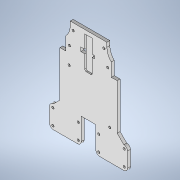
# Autodesk Inventor part: Основа робота
Saved by Autodesk Inventor 2020 (Build 240168000, 168)
## iProperties
Created: 2021-02-28
Part Number: Основа робота
Material: Типовые
Document SubType Name: Обычные детали
Designer: Антон
Density: 1 g/cm^3
Appearance: По умолчанию
Mass: 52.0111 g
Surface Area: 352.197 cm^2
Volume: 52.0111 cm^3
Sheet Metal Rule: По умолчанию
Author: Антон
Autodesk Inventor part; units mm, degrees
note: some values were not read from the file. Chosen so that the rebuilt part matches the saved one: direction of "Рельеф1".
ref_plane "YZ Plane" through (0, 0, 0) normal (1, 0, 0) x (0, 1, 0)
ref_plane "XZ Plane" through (0, 0, 0) normal (0, 1, 0) x (-1, 0, 0)
ref_plane "XY Plane" through (0, 0, 0) normal (0, 0, 1) x (1, 0, 0)
sketch "Эскиз1" plane through (0, 0, 0) normal (0, 0, 1) x (1, 0, 0)
  line L0 (0, 0) -> (39, 0)
  line L1 (39, 0) -> (39, 139.6)
  line L2 (39, 139.6) -> (0, 139.6)
  line L3 (0, 139.6) -> (0, 0)
  line L4 (0, 0) -> (-14.05, 0)
  line L5 (-14.05, 0) -> (-14.05, 30.3)
  line L6 (-14.05, 30.3) -> (0, 30.3)
  line L7 (0, 30.3) -> (0, 0)
  line L8 (-14.05, 0) -> (-9.5, 0)
  line L9 (-9.5, 0) -> (-9.5, 4.55)
  line L10 (-9.5, 4.55) -> (-9.5, 25.75)
  circle A0 centre (-9.5, 25.75) radius 1.6
  circle A1 centre (-9.5, 4.55) radius 1.6
  line L11 (39, 0) -> (29, 0)
  line L12 (29, 0) -> (29, 35)
  line L13 (29, 35) -> (39, 35)
  line L14 (39, 35) -> (39, 0)
  line L15 (29, 4.55) -> (25, 4.55)
  line L16 (29, 25.75) -> (25, 25.75)
  circle A2 centre (25, 25.75) radius 1.6
  circle A3 centre (25, 4.55) radius 1.6
  line L17 (39, 139.6) -> (39, 130.4)
  line L18 (39, 130.4) -> (18, 130.4)
  circle A4 centre (18, 130.4) radius 1.6
  line L19 (39, 139.6) -> (34, 139.6)
  line L20 (34, 139.6) -> (18, 139.6)
  line L21 (25, 25.75) -> (25, 4.55)
  circle A5 centre (12.95, 110.25) radius 1.6
  line L22 (0, 139.6) -> (14, 139.6)
  line L23 (14, 139.6) -> (14, 119.25)
  line L24 (14, 119.25) -> (0, 119.25)
  line L25 (0, 119.25) -> (0, 139.6)
  line L26 (0, 119.25) -> (8, 119.25)
  line L27 (8, 119.25) -> (8, 101.25)
  line L28 (8, 101.25) -> (0, 101.25)
  line L29 (0, 101.25) -> (0, 119.25)
  point P0 (0, 30.3)
  point P1 (29, 0)
  point P2 (39, 35)
  point P3 (0, 182.1)
  point P4 (25, 15.15)
  point P5 (-9.5, 15.15)
  point P6 (0, 119.25)
  point P7 (8, 119.25)
  point P8 (0, 101.25)
  dimension "d0" = 39
  dimension "d1" = 139.6
  dimension "d191" = 14.05
  dimension "d192" = 30.3
  dimension "d207" = 4.55
  dimension "d208" = 4.55
  dimension "d209" = 21.2
  dimension "d210" = 10
  dimension "d211" = 35
  dimension "d215" = 4
  dimension "d290" = 3.2
  dimension "d309" = 21
  dimension "d311" = 3.2
  dimension "d325" = 9.2
  dimension "d387" = 21.2
  dimension "d418" = 4.55
  dimension "d419" = 12.95
  dimension "d420" = 29.35
  dimension "d421" = 3.2
  dimension "d424" = 14
  dimension "d425" = 20.35
  dimension "d427" = 8
  dimension "d428" = 18
  constraints: 60 end point, 11 parallel, 8 perpendicular, 7 horizontal, 6 centre point, 6 point on line, 5 coincident, 3 equal radius, 2 midpoint, 1 collinear, 1 horizontal alignment, 1 vertical
  measures "d0" distance of L2.end L1.end
  measures "d1" distance of L1.end L0.end
  measures "d191" distance of L5.end L6.end
  measures "d192" distance of L4.end L5.end
  measures "d207" distance of L4.end L8.end
  measures "d208" distance of L8.end L9.end
  measures "d209" distance of L9.end L10.end
  measures "d210" distance of L12.end L13.end
  measures "d211" distance of L11.end L12.end
  measures "d215" distance of L16.start L16.end
  measures "d290" diameter of A2
  measures "d309" distance of L17.end L18.end
  measures "d311" diameter of A4
  measures "d325" distance from line of L19.end L18
  measures "d387" distance of L21.end L21.start
  measures "d418" distance from line of L0 L15.end
  measures "d419" distance from line of L3 A5.centre
  measures "d420" distance from line of L2 A5.centre
  measures "d421" diameter of A5
  measures "d424" distance of L23.end L24.end
  measures "d425" distance of L22.end L23.end
  measures "d427" distance of L27.end L28.end
  measures "d428" distance of L26.end L27.end
extrude "Выдавливание1" add sketch "Эскиз1" along normal blind 4 contours L3 L28 L27 L24 L23 L2 L1 L13 L12 L16 A2 L21 A3 L15 L0 | L4 L5 L6 L3 | L15 A3 L21 A2 L16 L12
mirror "Зеркальное отражение1" about plane through (39, 35, 0) normal (1, 0, 0) of "Выдавливание1"
sketch "Эскиз18" plane through (0, 0, 4) normal (0, 0, 1) x (1, 0, 0)
  line L0 (39, 139.6) -> (39, 86.75)
  line L1 (39, 86.75) -> (12.6, 86.75)
  line L2 (39, 86.75) -> (39, 41.05)
  line L3 (39, 41.05) -> (67.8, 41.05)
  line L4 (14, 139.6) -> (64, 139.6) projected
  point P0 (-4.55, 159.6)
  point P1 (82.55, 159.6)
  point P2 (0, 139.6)
  point P3 (78, 139.6)
  dimension "d218" = 52.85
  dimension "d220" = 26.4
  dimension "d221" = 45.7
  dimension "d222" = 28.8
  constraints: 8 end point, 2 horizontal, 2 vertical, 2 other
  measures "d218" distance of L0.start L0.end
  measures "d220" distance of L0.end L1.end
  measures "d221" distance of L0.end L2.end
  measures "d222" distance of L2.end L3.end
hole "Отверстие10" at (12.6, 86.75, 4) at (67.8, 41.05, 4) direction (0, 0, -1) diameter 3.2 end through all
fillet "Сопряжение2" radius 5.05 6 edges at (-14.05, 30.3, 2) (-14.05, 0, 2) (29, 0, 2) (49, 0, 2) (92.05, 0, 2) (92.05, 30.3, 2)
sketch "Эскиз19" plane through (0, 0, 0) normal (0, 0, -1) x (-1, 0, 0)
  line L0 (-14, 139.6) -> (-64, 139.6) projected
  circle A0 centre (-12.6, 86.75) radius 1.6 projected
  circle A1 centre (-12.6, 86.75) radius 1.6 projected
  line L1 (-15.4, 88.3666) -> (-12.6, 89.9832)
  line L2 (-12.6, 89.9832) -> (-9.8, 88.3666)
  line L3 (-9.8, 88.3666) -> (-9.8, 85.1334)
  line L4 (-9.8, 85.1334) -> (-12.6, 83.5168)
  line L5 (-12.6, 83.5168) -> (-15.4, 85.1334)
  line L6 (-15.4, 85.1334) -> (-15.4, 88.3666)
  line L7 (0, 101.25) -> (0, 30.3) projected
  point P0 (0, 139.6)
  point P1 (-78, 139.6)
  point P2 (0, 119.25)
  dimension "d423" = 5.6
  constraints: 12 end point, 1 coincident, 1 parallel, 13 other
  measures "d423" distance between parallel lines of L3 L6
extrude "Выдавливание7" cut sketch "Эскиз19" against normal blind 2.6 contours A0 | L1 L2 L3 L4 L5 L6
chamfer "Фаска1" distance 9 angle 45 2 edges at (0, 30.3, 2) (78, 30.3, 2)
sketch "Эскиз21" plane through (0, 0, 4) normal (0, 0, 1) x (1, 0, 0)
  line L0 (39, 139.6) -> (39, 134.4)
  line L1 (44.05, 134.4) -> (33.95, 134.4)
  line L2 (33.95, 134.4) -> (33.95, 90.75)
  line L3 (33.95, 90.75) -> (44.05, 90.75)
  line L4 (44.05, 90.75) -> (44.05, 134.4)
  line L5 (42, 92.8) -> (36, 92.8) construction
  line L6 (42, 90.75) -> (36, 90.75)
  line L7 (36, 94.85) -> (42, 94.85)
  arc A0 (42, 90.75) -> (42, 94.85) centre (42, 92.8) ccw
  arc A1 (36, 94.85) -> (36, 90.75) centre (36, 92.8) ccw
  line L8 (14, 139.6) -> (64, 139.6) projected
  point P0 (0, 0)
  point P1 (39, 92.8)
  point P2 (33.95, 92.8)
  point P3 (42, 90.75)
  point P4 (44.05, 92.8)
  point P5 (-4.55, 159.6)
  point P6 (82.55, 159.6)
  point P7 (0, 139.6)
  point P8 (78, 139.6)
  dimension "d297" = 10.1
  dimension "d298" = 43.65
  dimension "d299" = 5.2
  dimension "d307" = 4.1
  constraints: 18 end point, 6 tangent, 4 point on circle, 3 parallel, 2 centre point, 2 midpoint, 2 perpendicular, 1 collinear, 1 horizontal, 1 vertical, 2 other
  measures "d297" distance of L3.end L2.end
  measures "d298" distance of L2.end L1.end
  measures "d299" distance of L0.start L0.end
  measures "d307" distance between parallel lines of L3 L7
extrude "Выдавливание9" cut sketch "Эскиз21" against normal blind 2 contours L4 A0 L7 A1 L2 L1 | A0 L3 A1 L7
sketch "Эскиз25" plane through (0, 0, 0) normal (0, 0, -1) x (-1, 0, 0)
  circle A0 centre (-25, 25.75) radius 1.6 projected
  circle A1 centre (-25, 4.55) radius 1.6 projected
  circle A2 centre (9.5, 25.75) radius 1.6 projected
  circle A3 centre (9.5, 4.55) radius 1.6 projected
  circle A4 centre (-53, 25.75) radius 1.6 projected
  circle A5 centre (-53, 4.55) radius 1.6 projected
  circle A6 centre (-87.5, 4.55) radius 1.6 projected
  circle A7 centre (-87.5, 25.75) radius 1.6 projected
  circle A8 centre (-67.8, 41.05) radius 1.6 projected
  circle A9 centre (-12.6, 86.75) radius 1.6 projected
  circle A10 centre (-18, 130.4) radius 1.6 projected
  circle A11 centre (-60, 130.4) radius 1.6 projected
  circle A12 centre (-65.05, 110.25) radius 1.6 projected
  circle A13 centre (-12.95, 110.25) radius 1.6 projected
  circle A14 centre (-65.05, 110.25) radius 1.6 projected
  circle A15 centre (-12.95, 110.25) radius 1.6 projected
  point P0 (0, 0)
  constraints: 14 coincident
pattern_sketch "Массив по эскизу1" of "Выдавливание7" from (12.6, 86.75, 0) copies at (25, 25.75, 0) at (25, 4.55, 0) at (-9.5, 25.75, 0) at (-9.5, 4.55, 0) at (53, 25.75, 0) at (53, 4.55, 0) at (87.5, 4.55, 0) at (87.5, 25.75, 0) at (67.8, 41.05, 0) at (18, 130.4, 0) at (60, 130.4, 0) at (65.05, 110.25, 0) at (12.95, 110.25, 0)
sketch "Эскиз29" plane through (0, 0, 4) normal (0, 0, 1) x (1, 0, 0)
  line L0 (47.05, 111.6) -> (44.05, 111.6)
  line L1 (44.05, 111.6) -> (44.05, 115.6)
  line L2 (44.05, 115.6) -> (47.05, 115.6)
  line L3 (47.05, 115.6) -> (47.05, 111.6)
  line L4 (44.05, 134.4) -> (44.05, 92.8) projected
  line L5 (33.95, 110.85) -> (28.45, 110.85)
  line L6 (28.45, 110.85) -> (28.45, 116.35)
  line L7 (28.45, 116.35) -> (33.95, 116.35)
  line L8 (33.95, 116.35) -> (33.95, 110.85)
  line L9 (33.95, 92.8) -> (33.95, 134.4) projected
  point P0 (0, 0)
  point P1 (44.05, 113.6)
  point P2 (44.05, 136.615)
  point P3 (33.95, 113.6)
  point P4 (33.95, 136.615)
  dimension "d405" = 3
  dimension "d406" = 4
  dimension "d407" = 5.5
  dimension "d408" = 5.5
  constraints: 16 end point, 4 midpoint, 4 parallel, 2 horizontal, 2 perpendicular
  measures "d405" distance of L1.end L2.end
  measures "d406" distance of L0.end L1.end
  measures "d407" distance of L5.start L5.end
  measures "d408" distance of L5.end L6.end
extrude "Выдавливание13" cut sketch "Эскиз29" against normal through all
fillet "Сопряжение10" radius 20.35 2 edges at (64, 119.25, 2) (14, 119.25, 2)
sketch "Эскиз31" plane through (0, 0, 0) normal (0, 0, -1) x (-1, 0, 0)
  line L0 (-51.5, 80.5569) -> (-26.5, 80.5569) construction
  line L1 (-26.5, 80.5569) -> (-26.5, 59.9931) construction
  line L2 (-26.5, 59.9931) -> (-51.5, 59.9931) construction
  line L3 (-51.5, 59.9931) -> (-51.5, 80.5569) construction
  line L4 (-29, 35) -> (-49, 35) projected
  line L5 (-78, 101.25) -> (-78, 39.3) projected
  line L6 (0, 101.25) -> (0, 39.3) projected
  line L7 (-78, 101.25) -> (0, 101.25)
  line L8 (0, 101.25) -> (0, 39.3)
  line L9 (0, 39.3) -> (-78, 39.3)
  line L10 (-78, 39.3) -> (-78, 101.25)
  line L11 (-39, 101.25) -> (-39, 39.3)
  line L12 (-51.5, 70.275) -> (-26.5, 70.275)
  line L13 (-47.3655, 75.4476) -> (-45.8166, 80.22)
  line L14 (-45.8166, 80.22) -> (-44.6499, 80.22)
  line L15 (-44.6499, 80.22) -> (-46.8475, 74.12)
  line L16 (-46.8475, 74.12) -> (-47.8734, 74.12)
  line L17 (-47.8734, 74.12) -> (-50.061, 80.22)
  line L18 (-50.061, 80.22) -> (-48.8993, 80.22)
  line L19 (-48.8993, 80.22) -> (-47.3655, 75.4476)
  line L20 (-42.9803, 74.12) -> (-43.9962, 74.12)
  line L21 (-43.9962, 74.12) -> (-43.9962, 78.651)
  line L22 (-43.9962, 78.651) -> (-42.9803, 78.651)
  line L23 (-42.9803, 78.651) -> (-42.9803, 74.12)
  spline S0 degree 2 poles (-44.0615, 79.8277) (-44.0615, 80.059) (-43.7648, 80.3708) (-43.2117, 80.3708) (-42.9099, 80.059) (-42.9099, 79.8277) knots 0 0 0 1 2 3 4 4 4
  spline S1 degree 2 poles (-42.9099, 79.8277) (-42.9099, 79.5964) (-43.2117, 79.2896) (-43.7648, 79.2896) (-44.0615, 79.5964) (-44.0615, 79.8277) knots 0 0 0 1 2 3 4 4 4
  spline S2 degree 2 poles (-42.0601, 76.4282) (-42.0601, 77.092) (-41.532, 78.1632) (-40.5765, 78.7365) (-39.958, 78.7365) knots 0 0 0 1 2 3 3 3
  spline S3 degree 2 poles (-39.958, 78.7365) (-39.0427, 78.7365) (-37.8962, 77.5547) (-37.8509, 76.5791) knots 0 0 0 1 2 2 2
  line L24 (-37.8509, 76.5791) -> (-37.8459, 76.3377)
  spline S4 degree 2 poles (-37.8459, 76.3377) (-37.8459, 75.6689) (-38.3639, 74.6128) (-39.3244, 74.0345) (-39.9479, 74.0345) knots 0 0 0 1 2 3 3 3
  spline S5 degree 2 poles (-39.9479, 74.0345) (-40.9085, 74.0345) (-42.0601, 75.3118) (-42.0601, 76.3779) knots 0 0 0 1 2 2 2
  line L25 (-42.0601, 76.3779) -> (-42.0601, 76.4282)
  spline S6 degree 2 poles (-41.0442, 76.3427) (-41.0442, 75.6437) (-40.4659, 74.8491) (-39.435, 74.8491) (-38.8617, 75.6538) (-38.8617, 76.4282) knots 0 0 0 1 2 3 4 4 4
  spline S7 degree 2 poles (-38.8617, 76.4282) (-38.8617, 77.1172) (-39.4501, 77.9218) (-39.958, 77.9218) knots 0 0 0 1 2 2 2
  spline S8 degree 2 poles (-39.958, 77.9218) (-40.4559, 77.9218) (-41.0442, 77.1272) (-41.0442, 76.3427) knots 0 0 0 1 2 2 2
  line L26 (-35.9047, 74.12) -> (-36.9206, 74.12)
  line L27 (-36.9206, 74.12) -> (-36.9206, 80.5569)
  line L28 (-36.9206, 80.5569) -> (-35.9047, 80.5569)
  line L29 (-35.9047, 80.5569) -> (-35.9047, 74.12)
  spline S9 degree 2 poles (-32.8019, 74.0345) (-33.7675, 74.0345) (-34.9694, 75.2565) (-34.9694, 76.2673) knots 0 0 0 1 2 2 2
  line L30 (-34.9694, 76.2673) -> (-34.9694, 76.393)
  spline S10 degree 2 poles (-34.9694, 76.393) (-34.9694, 77.0719) (-34.4464, 78.143) (-33.5009, 78.7365) (-32.9176, 78.7365) knots 0 0 0 1 2 3 3 3
  spline S11 degree 2 poles (-32.9176, 78.7365) (-31.9923, 78.7365) (-30.9815, 77.5547) (-30.9815, 76.4785) knots 0 0 0 1 2 2 2
  line L31 (-30.9815, 76.4785) -> (-30.9815, 76.0661)
  line L32 (-30.9815, 76.0661) -> (-33.9435, 76.0661)
  spline S12 degree 2 poles (-33.9435, 76.0661) (-33.8982, 75.5029) (-33.2394, 74.8491) (-32.7416, 74.8491) knots 0 0 0 1 2 2 2
  spline S13 degree 2 poles (-32.7416, 74.8491) (-32.0426, 74.8491) (-31.6, 75.4124) knots 0 0 0 1 1 1
  line L33 (-31.6, 75.4124) -> (-31.0519, 74.8894)
  spline S14 degree 2 poles (-31.0519, 74.8894) (-31.3235, 74.482) (-32.2337, 74.0345) (-32.8019, 74.0345) knots 0 0 0 1 2 2 2
  spline S15 degree 2 poles (-32.9226, 77.9218) (-33.34, 77.9218) (-33.858, 77.3334) (-33.9284, 76.8104) knots 0 0 0 1 2 2 2
  line L34 (-33.9284, 76.8104) -> (-31.9873, 76.8104)
  line L35 (-31.9873, 76.8104) -> (-31.9873, 76.8858)
  spline S16 degree 2 poles (-31.9873, 76.8858) (-32.0225, 77.3988) (-32.5002, 77.9218) (-32.9226, 77.9218) knots 0 0 0 1 2 2 2
  line L36 (-28.9197, 79.7523) -> (-28.9197, 78.651)
  line L37 (-28.9197, 78.651) -> (-28.1201, 78.651)
  line L38 (-28.1201, 78.651) -> (-28.1201, 77.8966)
  line L39 (-28.1201, 77.8966) -> (-28.9197, 77.8966)
  line L40 (-28.9197, 77.8966) -> (-28.9197, 75.3671)
  spline S17 degree 2 poles (-28.9197, 75.3671) (-28.9197, 75.1056) (-28.7135, 74.8743) (-28.452, 74.8743) knots 0 0 0 1 2 2 2
  spline S18 degree 2 poles (-28.452, 74.8743) (-28.276, 74.8743) (-28.0949, 74.9145) knots 0 0 0 1 1 1
  line L41 (-28.0949, 74.9145) -> (-28.0949, 74.13)
  spline S19 degree 2 poles (-28.0949, 74.13) (-28.4419, 74.0345) (-28.7638, 74.0345) knots 0 0 0 1 1 1
  spline S20 degree 2 poles (-28.7638, 74.0345) (-29.9355, 74.0345) (-29.9355, 75.3269) knots 0 0 0 1 1 1
  line L42 (-29.9355, 75.3269) -> (-29.9355, 77.8966)
  line L43 (-29.9355, 77.8966) -> (-30.6798, 77.8966)
  line L44 (-30.6798, 77.8966) -> (-30.6798, 78.651)
  line L45 (-30.6798, 78.651) -> (-29.9355, 78.651)
  line L46 (-29.9355, 78.651) -> (-29.9355, 79.7523)
  line L47 (-29.9355, 79.7523) -> (-28.9197, 79.7523)
  line L48 (-47.6823, 69.6792) -> (-45.9272, 65.0024)
  line L49 (-45.9272, 65.0024) -> (-44.1722, 69.6792)
  line L50 (-44.1722, 69.6792) -> (-42.7993, 69.6792)
  line L51 (-42.7993, 69.6792) -> (-42.7993, 63.5792)
  line L52 (-42.7993, 63.5792) -> (-43.8554, 63.5792)
  line L53 (-43.8554, 63.5792) -> (-43.8554, 65.5908)
  line L54 (-43.8554, 65.5908) -> (-43.7498, 68.2812)
  line L55 (-43.7498, 68.2812) -> (-45.5501, 63.5792)
  line L56 (-45.5501, 63.5792) -> (-46.3094, 63.5792)
  line L57 (-46.3094, 63.5792) -> (-48.1098, 68.2762)
  line L58 (-48.1098, 68.2762) -> (-48.0042, 65.5908)
  line L59 (-48.0042, 65.5908) -> (-48.0042, 63.5792)
  line L60 (-48.0042, 63.5792) -> (-49.0602, 63.5792)
  line L61 (-49.0602, 63.5792) -> (-49.0602, 69.6792)
  line L62 (-49.0602, 69.6792) -> (-47.6823, 69.6792)
  line L63 (-40.1692, 65.5204) -> (-40.6218, 65.0577)
  line L64 (-40.6218, 65.0577) -> (-40.6218, 63.5792)
  line L65 (-40.6218, 63.5792) -> (-41.6427, 63.5792)
  line L66 (-41.6427, 63.5792) -> (-41.6427, 70.0162)
  line L67 (-41.6427, 70.0162) -> (-40.6218, 70.0162)
  line L68 (-40.6218, 70.0162) -> (-40.6218, 66.2998)
  line L69 (-40.6218, 66.2998) -> (-40.305, 66.6971)
  line L70 (-40.305, 66.6971) -> (-39.0528, 68.1102)
  line L71 (-39.0528, 68.1102) -> (-37.8308, 68.1102)
  line L72 (-37.8308, 68.1102) -> (-39.5155, 66.2194)
  line L73 (-39.5155, 66.2194) -> (-37.6498, 63.5792)
  line L74 (-37.6498, 63.5792) -> (-38.8265, 63.5792)
  line L75 (-38.8265, 63.5792) -> (-40.1692, 65.5204)
  spline S21 degree 2 poles (-36.5333, 64.6504) (-36.2517, 64.6504) (-35.9399, 64.3285) (-35.9399, 64.0871) knots 0 0 0 1 2 2 2
  spline S22 degree 2 poles (-35.9399, 64.0871) (-35.9399, 63.8458) (-36.2517, 63.534) (-36.5333, 63.534) knots 0 0 0 1 2 2 2
  spline S23 degree 2 poles (-36.5333, 63.534) (-36.8049, 63.534) (-37.1268, 63.8458) (-37.1268, 64.3285) (-36.815, 64.6504) (-36.5333, 64.6504) knots 0 0 0 1 2 3 4 4 4
  line L76 (-31.419, 63.5792) -> (-32.4751, 63.5792)
  line L77 (-32.4751, 63.5792) -> (-32.4751, 69.6792)
  line L78 (-32.4751, 69.6792) -> (-31.419, 69.6792)
  line L79 (-31.419, 69.6792) -> (-31.419, 63.5792)
  line L80 (-29.0001, 63.5792) -> (-30.0562, 63.5792)
  line L81 (-30.0562, 63.5792) -> (-30.0562, 69.6792)
  line L82 (-30.0562, 69.6792) -> (-29.0001, 69.6792)
  line L83 (-29.0001, 69.6792) -> (-29.0001, 63.5792)
  point P0 (0, 0)
  point P1 (-39, 70.275)
  dimension "d430" = 25
  constraints: 12 end point, 6 midpoint, 2 parallel, 1 horizontal, 1 perpendicular, 2 other
  measures "d430" distance of L12.start L12.end
emboss "Рельеф1" sketch "Эскиз31" operation cut depth 0.5 direction (0, 0, 1) contours S3 L24 S4 L11 S6 S7 | L11 S7 S8 S6 S4 S5 L25 S2 S3 | L75 L63 L64 L65 L66 L67 L68 L69 L70 L71 L11 L72 L73 | L11 L73 L74 L75 | L11 L71 L72 | L13 L14 L15 L16 L17 L18 L19 | L20 L21 L22 L23 | S0 S1 | L26 L27 L28 L29 | S9 L30 S10 S11 L31 L32 S12 S13 L33 S14 | L36 L37 L38 L39 L40 S17 S18 L41 S19 S20 L42 L43 L44 L45 L46 L47 | L48 L49 L50 L51 L52 L53 L54 L55 L56 L57 L58 L59 L60 L61 L62 | S21 S22 S23 | L76 L77 L78 L79 | L80 L81 L82 L83
equation "\"Радиус_гибки\" = Толщина"
equation "\"Ширина_просечки\" = Толщина"
equation "\"Глубина_просечки\" = 0.5 * Толщина"
equation "\"Размер_просечки\" = 4 * Толщина"
equation "\"Мин_остаток\" = 2 * Толщина"
equation "\"Радиус_перехода\" = Радиус_гибки"
equation "\"Радиус_Якоби\" = Толщина"
equation "\"Размер_зазора\" = Толщина"
equation "\"Гайка_М3_з\" = 5.6"
equation "\"d130\" = 5.6"
equation "\"Толщина\" = 0.5"
